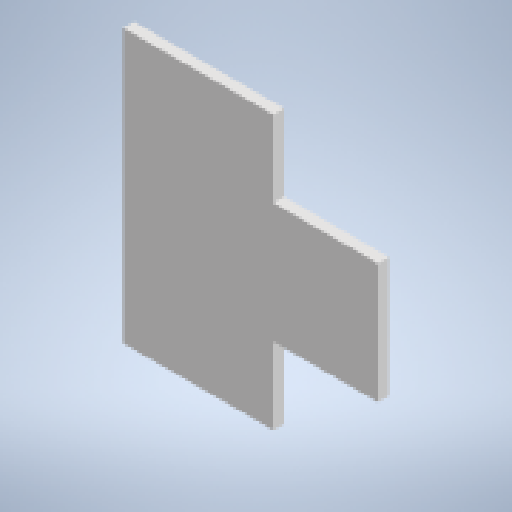
# Autodesk Inventor part: PCB_BYK
Saved by Autodesk Inventor 2023 (Build 270158000, 158)
## iProperties
Created: 2023-12-19
Part Number: PCB_BYK
Material: Ogólny
Document SubType Name: Modeling
Designer: Kamil
Density: 1 g/cm^3
Appearance: Domyślna
Author: Kamil
Autodesk Inventor part; units mm, degrees
ref_plane "YZ Plane" through (0, 0, 0) normal (1, 0, 0) x (0, 1, 0)
ref_plane "XZ Plane" through (0, 0, 0) normal (0, 1, 0) x (-1, 0, 0)
ref_plane "XY Plane" through (0, 0, 0) normal (0, 0, 1) x (1, 0, 0)
sketch "Szkic1" plane through (0, 0, 0) normal (0, 0, 1) x (1, 0, 0)
  line L0 (7, 11) -> (-7, 11) projected
  line L1 (-7, 11) -> (-7, -11) projected
  line L2 (-7, -11) -> (7, -11) projected
  line L3 (7, -11) -> (7, 11) projected
  line L4 (-39.6549, 25) -> (-39.6549, -25) projected
  line L5 (-7, -25) -> (-39.6549, -25) projected
  line L6 (-7, -25) -> (-7, -11) projected
  line L7 (-7, -11) -> (7, -11) projected
  line L8 (7, 11) -> (7, -11) projected
  line L9 (7, 11) -> (-7, 11) projected
  line L10 (-7, 11) -> (-7, 25) projected
  line L11 (-39.6549, 25) -> (-7, 25) projected
  line L12 (-12.1691, 22.3198) -> (-12.1691, 17.3208) projected
  line L13 (-12.1691, -19.1802) -> (-12.1691, -24.1792) projected
  line L14 (-12.1691, 22.3198) -> (-12.1691, 25)
  line L15 (-12.1691, 17.3208) -> (-12.1691, -19.1802)
  line L16 (-12.1691, -24.1792) -> (-12.1691, -25)
  line L17 (-7, 11) -> (-12.1691, 11)
  line L18 (-7, -11) -> (-12.1691, -11)
  point P0 (0, 0)
  constraints: 10 end point, 5 point on line, 2 perpendicular, 1 collinear, 1 parallel
extrude "Wyciągnięcie proste1" add sketch "Szkic1" along normal blind 2 contours L3 L2 L1 L0 | L1 L18 L15 L17 | L15 L13 L16 L5 L4 L11 L14 L12
sketch "Szkic2" plane through (-39.6549, 25, 0) normal (0, 1, 0) x (1, 0, 0)
  line L0 (3.2737, -2) -> (-1.2456, 12.15) projected
  line L1 (27.4857, 0) -> (0, 0) projected
  line L2 (0, 0) -> (0, -2) projected
  line L3 (27.4857, -2) -> (0, -2) projected
  line L4 (27.4857, 0) -> (27.4857, -2) projected
  line L5 (3.2737, -2) -> (3.2737, 0)
  point P0 (39.6549, 0)
  constraints: 3 point on line, 2 end point, 1 vertical
extrude "Wyciągnięcie proste2" cut sketch "Szkic2" against normal through all contours L3 L2 L1 L0 | L0 L1 L5
